Autodesk Fusion 360 part; units mm, degrees
(part 6 of 25)
  arc A2041 (23.4513, 13.1318) -> (23.4513, 13.1826) centre (23.4513, 13.1572) ccw
  line L640 (23.4513, 12.5081) -> (23.1267, 12.5081)
  arc A2042 (23.1521, 13.1572) -> (23.1013, 13.1572) centre (23.1267, 13.1572) ccw
  arc A2043 (25.2656, 11.9888) -> (25.3164, 11.9888) centre (25.291, 11.9888) ccw
  arc A2044 (26.4688, 12.2484) -> (26.7285, 11.9888) centre (26.7285, 12.2485) ccw
  arc A2045 (25.9147, 11.9888) -> (25.9655, 11.9888) centre (25.9401, 11.9888) ccw
  arc A2046 (21.1404, 12.6633) -> (21.1404, 12.6125) centre (21.1404, 12.6379) ccw
  line L641 (22.131, 13.1572) -> (22.6503, 13.1572)
  line L642 (25.291, 13.1572) -> (25.9401, 11.9888)
  arc A2047 (23.1267, 12.5335) -> (23.1267, 12.4827) centre (23.1267, 12.5081) ccw
  arc A2048 (22.131, 13.1826) -> (22.131, 13.1318) centre (22.131, 13.1572) ccw
  line L643 (23.1267, 13.1572) -> (23.4513, 13.1572)
  arc A2049 (23.4513, 12.5081) -> (23.4513, 13.1572) centre (23.4513, 12.8327) ccw
  arc A2050 (22.1564, 13.1572) -> (22.1056, 13.1572) centre (22.131, 13.1572) ccw
  arc A2051 (24.822, 13.1318) -> (24.822, 13.1826) centre (24.822, 13.1572) ccw
  arc A2052 (57.8335, 39.6198) -> (57.8335, 39.569) centre (57.8335, 39.5944) ccw
  arc A2053 (27.9843, 11.9634) -> (27.9843, 12.0142) centre (27.9843, 11.9888) ccw
  arc A2054 (25.9655, 13.1572) -> (25.9147, 13.1572) centre (25.9401, 13.1572) ccw
  arc A2055 (23.5389, 12.5194) -> (23.4934, 12.4967) centre (23.5162, 12.5081) ccw
  arc A2056 (23.4513, 12.4827) -> (23.4513, 12.5335) centre (23.4513, 12.5081) ccw
  arc A2057 (23.4513, 12.5335) -> (23.4513, 12.4827) centre (23.4513, 12.5081) ccw
  arc A2058 (26.7285, 13.1318) -> (26.7285, 13.1826) centre (26.7285, 13.1572) ccw
  arc A2059 (22.5205, 12.6125) -> (22.5205, 12.6633) centre (22.5205, 12.6379) ccw
  line L644 (24.3027, 12.6379) -> (24.6922, 12.6379)
  arc A2060 (24.3027, 12.0142) -> (24.3027, 11.9634) centre (24.3027, 11.9888) ccw
  arc A2061 (24.6922, 12.6125) -> (24.6922, 12.6633) centre (24.6922, 12.6379) ccw
  arc A2062 (22.6503, 13.1318) -> (22.6503, 13.1826) centre (22.6503, 13.1572) ccw
  line L645 (22.6503, 11.9888) -> (22.131, 11.9888)
  line L646 (23.7758, 11.9888) -> (23.5162, 12.5081)
  arc A2063 (27.465, 12.0142) -> (27.465, 11.9634) centre (27.465, 11.9888) ccw
  line L647 (23.1267, 11.9888) -> (23.1267, 13.1572)
  line L648 (27.465, 11.9888) -> (27.465, 13.1572)
  line L649 (21.1404, 12.6379) -> (21.6597, 12.6379)
  arc A2064 (26.7285, 11.9634) -> (26.7285, 12.0142) centre (26.7285, 11.9888) ccw
  line L650 (22.131, 12.6379) -> (22.5205, 12.6379)
  arc A2065 (26.4942, 12.2484) -> (26.4434, 12.2484) centre (26.4688, 12.2484) ccw
  arc A2066 (27.4904, 13.1572) -> (27.4396, 13.1572) centre (27.465, 13.1572) ccw
  arc A2067 (26.7285, 12.0142) -> (26.7285, 11.9634) centre (26.7285, 11.9888) ccw
  line L651 (24.3027, 11.9888) -> (24.3027, 13.1572)
  line L652 (22.131, 11.9888) -> (22.131, 13.1572)
  arc A2068 (23.1013, 11.9888) -> (23.1521, 11.9888) centre (23.1267, 11.9888) ccw
  arc A2069 (24.3027, 12.6633) -> (24.3027, 12.6125) centre (24.3027, 12.6379) ccw
  arc A2070 (22.131, 12.6633) -> (22.131, 12.6125) centre (22.131, 12.6379) ccw
  arc A2071 (23.1267, 13.1826) -> (23.1267, 13.1318) centre (23.1267, 13.1572) ccw
  arc A2072 (22.131, 12.0142) -> (22.131, 11.9634) centre (22.131, 11.9888) ccw
  line L653 (57.8984, 39.0751) -> (57.8984, 39.0102)
  line L654 (24.822, 11.9888) -> (24.3027, 11.9888)
  arc A2073 (23.4513, 13.1826) -> (23.4513, 13.1318) centre (23.4513, 13.1572) ccw
  arc A2074 (22.6503, 11.9634) -> (22.6503, 12.0142) centre (22.6503, 11.9888) ccw
  arc A2075 (24.3281, 13.1572) -> (24.2773, 13.1572) centre (24.3027, 13.1572) ccw
  line L655 (27.9843, 11.9888) -> (27.465, 11.9888)
  arc A2076 (25.3132, 13.1695) -> (25.2688, 13.1449) centre (25.291, 13.1572) ccw
  line L656 (26.9881, 11.9888) -> (26.7285, 11.9888)
  arc A2077 (19.2984, 13.1826) -> (19.2984, 13.1318) centre (19.2984, 13.1572) ccw
  arc A2078 (22.1056, 11.9888) -> (22.1564, 11.9888) centre (22.131, 11.9888) ccw
  arc A2079 (23.7531, 11.9774) -> (23.7985, 12.0002) centre (23.7758, 11.9888) ccw
  line L657 (25.291, 11.9888) -> (25.291, 13.1572)
  arc A2080 (24.2773, 11.9888) -> (24.3281, 11.9888) centre (24.3027, 11.9888) ccw
  line L658 (24.3027, 13.1572) -> (24.822, 13.1572)
  arc A2081 (19.2984, 10.5777) -> (19.2984, 10.6285) centre (19.2984, 10.6031) ccw
  arc A2082 (21.3939, 10.0584) -> (21.3939, 10.1092) centre (21.3939, 10.0838) ccw
  arc A2083 (20.0838, 10.3434) -> (20.033, 10.3434) centre (20.0584, 10.3434) ccw
  arc A2084 (21.0693, 11.2776) -> (21.0693, 11.2268) centre (21.0693, 11.2522) ccw
  line L659 (26.4688, 12.2484) -> (26.4688, 12.8976)
  arc A2085 (27.4396, 11.9888) -> (27.4904, 11.9888) centre (27.465, 11.9888) ccw
  arc A2086 (19.2984, 10.6031) -> (19.2984, 11.2522) centre (19.2984, 10.9277) ccw
  line L660 (21.0693, 10.0838) -> (21.0693, 11.2522)
  arc A2087 (21.0439, 10.0838) -> (21.0947, 10.0838) centre (21.0693, 10.0838) ccw
  line L661 (27.465, 12.6379) -> (27.8545, 12.6379)
  arc A2088 (26.4942, 12.8976) -> (26.4434, 12.8976) centre (26.4688, 12.8976) ccw
  arc A2089 (19.2984, 10.6285) -> (19.2984, 10.5777) centre (19.2984, 10.6031) ccw
  arc A2090 (27.465, 13.1826) -> (27.465, 13.1318) centre (27.465, 13.1572) ccw
  line L662 (21.0693, 10.7329) -> (21.3939, 10.7329)
  arc A2091 (20.0838, 10.9926) -> (20.033, 10.9926) centre (20.0584, 10.9926) ccw
  arc A2092 (21.3939, 11.2268) -> (21.3939, 11.2776) centre (21.3939, 11.2522) ccw
  arc A2093 (21.3939, 11.2776) -> (21.3939, 11.2268) centre (21.3939, 11.2522) ccw
  arc A2094 (21.3939, 10.1092) -> (21.3939, 10.0584) centre (21.3939, 10.0838) ccw
  arc A2095 (21.3939, 10.7583) -> (21.3939, 10.7075) centre (21.3939, 10.7329) ccw
  arc A2096 (26.4434, 12.2484) -> (26.4942, 12.2484) centre (26.4688, 12.2484) ccw
  arc A2097 (18.9738, 10.6285) -> (18.9738, 10.5777) centre (18.9738, 10.6031) ccw
  arc A2098 (20.3181, 11.2268) -> (20.3181, 11.2776) centre (20.3181, 11.2522) ccw
  arc A2099 (21.3939, 10.7075) -> (21.3939, 10.7583) centre (21.3939, 10.7329) ccw
  arc A2100 (20.3181, 11.2522) -> (20.0584, 10.9926) centre (20.3181, 10.9925) ccw
  arc A2101 (26.7285, 13.1572) -> (26.4688, 12.8976) centre (26.7285, 12.8975) ccw
  arc A2102 (27.465, 12.6633) -> (27.465, 12.6125) centre (27.465, 12.6379) ccw
  line L663 (21.0693, 11.2522) -> (21.3939, 11.2522)
  arc A2103 (21.0693, 10.7583) -> (21.0693, 10.7075) centre (21.0693, 10.7329) ccw
  arc A2104 (20.5777, 11.2268) -> (20.5777, 11.2776) centre (20.5777, 11.2522) ccw
  arc A2105 (19.2984, 11.2268) -> (19.2984, 11.2776) centre (19.2984, 11.2522) ccw
  line L664 (20.5777, 10.0838) -> (20.3181, 10.0838)
  arc A2106 (20.033, 10.9926) -> (20.0838, 10.9926) centre (20.0584, 10.9926) ccw
  arc A2107 (26.4434, 12.8976) -> (26.4942, 12.8976) centre (26.4688, 12.8976) ccw
  arc A2108 (20.3181, 10.1092) -> (20.3181, 10.0584) centre (20.3181, 10.0838) ccw
  arc A2109 (20.3181, 10.0584) -> (20.3181, 10.1092) centre (20.3181, 10.0838) ccw
  arc A2110 (20.5777, 10.0584) -> (20.5777, 10.1092) centre (20.5777, 10.0838) ccw
  arc A2111 (21.0947, 11.2522) -> (21.0439, 11.2522) centre (21.0693, 11.2522) ccw
  line L665 (19.2984, 10.6031) -> (18.9738, 10.6031)
  arc A2112 (26.9881, 13.1318) -> (26.9881, 13.1826) centre (26.9881, 13.1572) ccw
  line L666 (27.465, 13.1572) -> (27.9843, 13.1572)
  arc A2113 (21.0693, 10.1092) -> (21.0693, 10.0584) centre (21.0693, 10.0838) ccw
  arc A2114 (21.3939, 10.7583) -> (21.3939, 10.7075) centre (21.3939, 10.7329) ccw
  line L667 (20.0584, 10.3434) -> (20.0584, 10.9926)
  arc A2115 (20.0584, 10.3434) -> (20.3181, 10.0838) centre (20.3181, 10.3435) ccw
  arc A2116 (21.3939, 10.0838) -> (21.3939, 10.7329) centre (21.3939, 10.4084) ccw
  line L668 (21.3939, 10.0838) -> (21.0693, 10.0838)
  line L669 (26.7285, 13.1572) -> (26.9881, 13.1572)
  line L670 (18.9738, 11.2522) -> (19.2984, 11.2522)
  line L671 (25.9401, 11.9888) -> (25.9401, 13.1572)
  arc A2117 (20.3181, 11.2776) -> (20.3181, 11.2268) centre (20.3181, 11.2522) ccw
  arc A2118 (18.9992, 11.2522) -> (18.9484, 11.2522) centre (18.9738, 11.2522) ccw
  arc A2119 (18.9484, 10.0838) -> (18.9992, 10.0838) centre (18.9738, 10.0838) ccw
  line L672 (18.9738, 10.0838) -> (18.9738, 11.2522)
  arc A2120 (20.033, 10.3434) -> (20.0838, 10.3434) centre (20.0584, 10.3434) ccw
  arc A2121 (19.2984, 11.2776) -> (19.2984, 11.2268) centre (19.2984, 11.2522) ccw
  line L673 (20.3181, 11.2522) -> (20.5777, 11.2522)
  arc A2122 (18.9738, 11.2776) -> (18.9738, 11.2268) centre (18.9738, 11.2522) ccw
  arc A2123 (22.6314, 42.8554) -> (22.6822, 42.8554) centre (22.6568, 42.8554) ccw
  arc A2124 (21.3939, 10.7329) -> (21.3939, 11.2522) centre (21.3939, 10.9926) ccw
  arc A2125 (27.8545, 12.6125) -> (27.8545, 12.6633) centre (27.8545, 12.6379) ccw
  arc A2126 (27.9843, 13.1318) -> (27.9843, 13.1826) centre (27.9843, 13.1572) ccw
  arc A2127 (23.1761, 42.5704) -> (23.1761, 42.6212) centre (23.1761, 42.5958) ccw
  arc A2128 (22.9164, 43.7388) -> (22.9164, 43.7896) centre (22.9164, 43.7642) ccw
  arc A2129 (22.9814, 41.1988) -> (22.9814, 41.2496) centre (22.9814, 41.2242) ccw
  arc A2130 (22.6568, 41.2496) -> (22.6568, 41.1988) centre (22.6568, 41.2242) ccw
  arc A2131 (22.6568, 37.5412) -> (22.6568, 37.4904) centre (22.6568, 37.5158) ccw
  arc A2132 (22.6568, 40.0812) -> (22.6568, 40.0304) centre (22.6568, 40.0558) ccw
  arc A2133 (22.9814, 40.7303) -> (22.9814, 40.6795) centre (22.9814, 40.7049) ccw
  arc A2134 (22.6822, 43.5046) -> (22.6314, 43.5046) centre (22.6568, 43.5046) ccw
  line L674 (22.9164, 43.7642) -> (23.1761, 43.7642)
  arc A2135 (23.1761, 37.4904) -> (23.1761, 37.5412) centre (23.1761, 37.5158) ccw
  arc A2136 (22.6568, 38.1903) -> (22.6568, 38.1395) centre (22.6568, 38.1649) ccw
  arc A2137 (22.6822, 42.8554) -> (22.6314, 42.8554) centre (22.6568, 42.8554) ccw
  line L675 (22.6568, 37.5158) -> (22.6568, 38.6842)
  arc A2138 (72.1043, 51.3715) -> (72.0408, 51.3715) centre (72.0726, 51.3715) ccw
  arc A2139 (23.1761, 38.6588) -> (23.1761, 38.7096) centre (23.1761, 38.6842) ccw
  arc A2140 (72.3265, 52.2287) -> (72.3265, 52.2923) centre (72.3265, 52.2605) ccw
  line L676 (72.5805, 51.1175) -> (72.3265, 51.1175)
  arc A2141 (72.3265, 52.2605) -> (72.0725, 52.0065) centre (72.3265, 52.0065) ccw
  arc A2142 (73.0287, 51.1493) -> (73.0287, 51.0857) centre (73.0287, 51.1175) ccw
  line L677 (72.0725, 51.3715) -> (72.0725, 52.0065)
  arc A2143 (22.6314, 37.5158) -> (22.6822, 37.5158) centre (22.6568, 37.5158) ccw
  arc A2144 (72.0408, 52.0065) -> (72.1043, 52.0065) centre (72.0726, 52.0065) ccw
  arc A2145 (72.5805, 52.2287) -> (72.5805, 52.2923) centre (72.5805, 52.2605) ccw
  arc A2146 (73.6637, 51.0857) -> (73.6637, 51.1493) centre (73.6637, 51.1175) ccw
  arc A2147 (73.3145, 51.1175) -> (73.378, 51.1175) centre (73.3462, 51.1175) ccw
  arc A2148 (73.378, 52.2605) -> (73.3145, 52.2605) centre (73.3462, 52.2605) ccw
  arc A2149 (22.9164, 42.5704) -> (22.9164, 42.6212) centre (22.9164, 42.5958) ccw
  line L678 (22.6568, 40.7049) -> (22.9814, 40.7049)
  arc A2150 (22.9814, 40.0558) -> (22.9814, 40.7049) centre (22.9814, 40.3803) ccw
  line L679 (22.6568, 40.0558) -> (22.6568, 41.2242)
  line L680 (22.6568, 38.6842) -> (23.1761, 38.6842)
  arc A2151 (22.6822, 38.6842) -> (22.6314, 38.6842) centre (22.6568, 38.6842) ccw
  arc A2152 (72.1043, 52.0065) -> (72.0408, 52.0065) centre (72.0726, 52.0065) ccw
  arc A2153 (22.9814, 41.2496) -> (22.9814, 41.1988) centre (22.9814, 41.2242) ccw
  arc A2154 (22.9814, 40.7049) -> (22.9814, 41.2242) centre (22.9814, 40.9646) ccw
  arc A2155 (72.3265, 52.2923) -> (72.3265, 52.2287) centre (72.3265, 52.2605) ccw
  line L681 (22.6568, 38.1649) -> (23.0463, 38.1649)
  line L682 (73.0287, 52.0065) -> (73.3462, 52.2605)
  line L683 (23.1761, 42.5958) -> (22.9164, 42.5958)
  arc A2156 (22.9164, 42.6212) -> (22.9164, 42.5704) centre (22.9164, 42.5958) ccw
  arc A2157 (22.6314, 40.0558) -> (22.6822, 40.0558) centre (22.6568, 40.0558) ccw
  arc A2158 (22.6314, 43.5046) -> (22.6822, 43.5046) centre (22.6568, 43.5046) ccw
  arc A2159 (72.3265, 51.1493) -> (72.3265, 51.0857) centre (72.3265, 51.1175) ccw
  arc A2160 (72.5805, 51.0857) -> (72.5805, 51.1493) centre (72.5805, 51.1175) ccw
  line L684 (22.6568, 42.8554) -> (22.6568, 43.5046)
  arc A2161 (22.6568, 42.8554) -> (22.9164, 42.5958) centre (22.9164, 42.8554) ccw
  arc A2162 (22.9164, 43.7896) -> (22.9164, 43.7388) centre (22.9164, 43.7642) ccw
  arc A2163 (22.6568, 38.7096) -> (22.6568, 38.6588) centre (22.6568, 38.6842) ccw
  arc A2164 (22.6822, 41.2242) -> (22.6314, 41.2242) centre (22.6568, 41.2242) ccw
  line L685 (73.3462, 52.2605) -> (73.3462, 51.1175)
  arc A2165 (23.0463, 38.1395) -> (23.0463, 38.1903) centre (23.0463, 38.1649) ccw
  arc A2166 (72.0725, 51.3715) -> (72.3265, 51.1175) centre (72.3265, 51.3715) ccw
  arc A2167 (22.9814, 40.0812) -> (22.9814, 40.0304) centre (22.9814, 40.0558) ccw
  line L686 (22.9814, 40.0558) -> (22.6568, 40.0558)
  arc A2168 (22.9814, 40.7303) -> (22.9814, 40.6795) centre (22.9814, 40.7049) ccw
  line L687 (23.1761, 37.5158) -> (22.6568, 37.5158)
  arc A2169 (22.9164, 43.7642) -> (22.6568, 43.5046) centre (22.9164, 43.5046) ccw
  arc A2170 (23.1761, 43.7388) -> (23.1761, 43.7896) centre (23.1761, 43.7642) ccw
  arc A2171 (22.6568, 40.7303) -> (22.6568, 40.6795) centre (22.6568, 40.7049) ccw
  arc A2172 (22.9814, 40.0304) -> (22.9814, 40.0812) centre (22.9814, 40.0558) ccw
  line L688 (22.6568, 41.2242) -> (22.9814, 41.2242)
  arc A2173 (72.0408, 51.3715) -> (72.1043, 51.3715) centre (72.0726, 51.3715) ccw
  arc A2174 (22.9814, 40.6795) -> (22.9814, 40.7303) centre (22.9814, 40.7049) ccw
  arc A2175 (73.3661, 52.2357) -> (73.3264, 52.2853) centre (73.3463, 52.2605) ccw
  arc A2176 (73.0089, 52.0313) -> (73.0486, 51.9817) centre (73.0288, 52.0065) ccw
  line L689 (72.3265, 52.2605) -> (72.5805, 52.2605)
  arc A2177 (55.0545, 20.5422) -> (55.0545, 20.4788) centre (55.0545, 20.5105) ccw
  arc A2178 (56.106, 20.5105) -> (55.7567, 20.2565) centre (56.106, 20.1434) ccw
  arc A2179 (11.9697, 38.608) -> (12.0333, 38.608) centre (12.0015, 38.608) ccw
  arc A2180 (11.176, 38.9255) -> (10.8585, 38.608) centre (11.176, 38.608) ccw
  arc A2181 (11.9697, 38.2905) -> (12.0333, 38.2905) centre (12.0015, 38.2905) ccw
  arc A2182 (56.3917, 19.3358) -> (56.3917, 19.3992) centre (56.3917, 19.3675) ccw
  line L690 (12.0015, 38.2905) -> (10.8585, 38.2905)
  arc A2183 (11.1443, 40.0748) -> (11.1443, 40.1384) centre (11.1443, 40.1066) ccw
  arc A2184 (11.3871, 40.0355) -> (11.3459, 39.9872) centre (11.3665, 40.0114) ccw
  arc A2185 (12.0015, 38.608) -> (11.684, 38.9255) centre (11.684, 38.608) ccw
  arc A2186 (11.176, 38.8937) -> (11.176, 38.9573) centre (11.176, 38.9255) ccw
  arc A2187 (11.684, 38.9573) -> (11.684, 38.8937) centre (11.684, 38.9255) ccw
  line L691 (56.2965, 20.0025) -> (55.7567, 19.3675)
  arc A2188 (56.36, 20.2248) -> (56.4235, 20.2248) centre (56.3918, 20.2248) ccw
  arc A2189 (55.0545, 19.3358) -> (55.0545, 19.3992) centre (55.0545, 19.3675) ccw
  arc A2190 (55.3085, 19.3358) -> (55.3085, 19.3992) centre (55.3085, 19.3675) ccw
  arc A2191 (55.0545, 20.5105) -> (54.8005, 20.2565) centre (55.0545, 20.2565) ccw
  arc A2192 (55.7325, 19.3881) -> (55.7809, 19.3469) centre (55.7567, 19.3675) ccw
  arc A2193 (54.8323, 19.6215) -> (54.7687, 19.6215) centre (54.8005, 19.6215) ccw
  arc A2194 (56.106, 20.5422) -> (56.106, 20.4788) centre (56.106, 20.5105) ccw
  arc A2195 (55.0545, 19.3992) -> (55.0545, 19.3358) centre (55.0545, 19.3675) ccw
  arc A2196 (56.2746, 20.0255) -> (56.3184, 19.9795) centre (56.2965, 20.0025) ccw
  arc A2197 (56.4235, 20.2248) -> (56.36, 20.2247) centre (56.3918, 20.2248) ccw
  line L692 (54.8005, 19.6215) -> (54.8005, 20.2565)
  arc A2198 (54.7687, 19.6215) -> (54.8323, 19.6215) centre (54.8005, 19.6215) ccw
  arc A2199 (12.0015, 38.2587) -> (12.0015, 38.3223) centre (12.0015, 38.2905) ccw
  arc A2200 (55.0545, 20.4788) -> (55.0545, 20.5422) centre (55.0545, 20.5105) ccw
  arc A2201 (10.8585, 38.3223) -> (10.8585, 38.2587) centre (10.8585, 38.2905) ccw
  arc A2202 (11.176, 38.9573) -> (11.176, 38.8937) centre (11.176, 38.9255) ccw
  arc A2203 (11.1442, 40.1383) -> (11.1443, 40.0749) centre (11.1442, 40.1066) ccw
  arc A2204 (11.3665, 40.0114) -> (11.1443, 40.1066) centre (11.1444, 39.7998) ccw
  line L693 (55.0545, 20.5105) -> (55.3085, 20.5105)
  arc A2205 (54.7687, 20.2565) -> (54.8323, 20.2565) centre (54.8005, 20.2565) ccw
  arc A2206 (72.3265, 51.0857) -> (72.3265, 51.1493) centre (72.3265, 51.1175) ccw
  arc A2207 (56.2965, 20.0025) -> (56.3917, 20.2248) centre (56.0848, 20.2247) ccw
  arc A2208 (54.8005, 19.6215) -> (55.0545, 19.3675) centre (55.0545, 19.6215) ccw
  arc A2209 (55.7567, 19.3992) -> (55.7567, 19.3358) centre (55.7567, 19.3675) ccw
  arc A2210 (56.3207, 19.9819) -> (56.2723, 20.0231) centre (56.2965, 20.0025) ccw
  line L694 (12.0015, 39.4716) -> (12.0015, 40.1066)
  line L695 (10.8585, 38.2905) -> (10.8585, 38.608)
  arc A2211 (12.0333, 40.1066) -> (11.9697, 40.1066) centre (12.0015, 40.1066) ccw
  arc A2212 (10.8268, 39.8209) -> (10.8903, 39.8209) centre (10.8586, 39.8209) ccw
  arc A2213 (55.3085, 20.4788) -> (55.3085, 20.5422) centre (55.3085, 20.5105) ccw
  arc A2214 (10.8268, 38.608) -> (10.8903, 38.608) centre (10.8586, 38.608) ccw
  line L696 (55.7567, 19.3675) -> (56.3917, 19.3675)
  arc A2215 (11.1443, 40.1066) -> (10.8585, 39.8209) centre (11.1443, 39.8208) ccw
  arc A2216 (56.3917, 20.2248) -> (56.106, 20.5105) centre (56.106, 20.2248) ccw
  arc A2217 (43.9774, 31.3303) -> (44.017, 31.2807) centre (43.9972, 31.3055) ccw
  arc A2218 (10.8903, 38.608) -> (10.8268, 38.608) centre (10.8586, 38.608) ccw
  arc A2219 (56.106, 20.4788) -> (56.106, 20.5422) centre (56.106, 20.5105) ccw
  arc A2220 (11.684, 38.8937) -> (11.684, 38.9573) centre (11.684, 38.9255) ccw
  arc A2221 (12.0333, 38.608) -> (11.9697, 38.608) centre (12.0015, 38.608) ccw
  line L697 (55.3085, 19.3675) -> (55.0545, 19.3675)
  arc A2222 (11.3435, 39.9895) -> (11.3895, 40.0332) centre (11.3665, 40.0114) ccw
  arc A2223 (54.8323, 20.2565) -> (54.7687, 20.2565) centre (54.8005, 20.2565) ccw
  line L698 (11.176, 38.9255) -> (11.684, 38.9255)
  line L699 (73.0287, 51.1175) -> (73.6637, 51.1175)
  arc A2224 (11.9697, 39.4716) -> (12.0333, 39.4716) centre (12.0015, 39.4716) ccw
  line L700 (11.3665, 40.0114) -> (12.0015, 39.4716)
  arc A2225 (11.1027, 39.4414) -> (11.1223, 39.5018) centre (11.1125, 39.4716) ccw
  arc A2226 (10.8903, 39.8208) -> (10.8268, 39.8209) centre (10.8586, 39.8209) ccw
  arc A2227 (10.8268, 38.2905) -> (10.8903, 38.2905) centre (10.8586, 38.2905) ccw
  arc A2228 (55.7265, 20.2663) -> (55.7869, 20.2467) centre (55.7567, 20.2565) ccw
  line L701 (12.0015, 38.608) -> (12.0015, 38.2905)
  line L702 (71.2799, 44.5135) -> (71.2799, 44.0055)
  line L703 (42.3545, 30.4165) -> (42.1005, 30.9245)
  arc A2229 (42.037, 31.5278) -> (42.037, 31.5912) centre (42.037, 31.5595) ccw
  line L704 (42.037, 30.9245) -> (41.7195, 30.9245)
  arc A2230 (24.2264, 26.0668) -> (24.2264, 26.1303) centre (24.2264, 26.0985) ccw
  arc A2231 (41.7195, 30.9563) -> (41.7195, 30.8928) centre (41.7195, 30.9246) ccw
  arc A2232 (23.0505, 24.9555) -> (23.3045, 25.2095) centre (23.0505, 25.2095) ccw
  arc A2233 (23.0505, 24.9238) -> (23.0505, 24.9872) centre (23.0505, 24.9555) ccw
  arc A2234 (23.9724, 25.6223) -> (23.9724, 25.5588) centre (23.9724, 25.5906) ccw
  arc A2235 (43.4892, 30.3848) -> (43.4892, 30.4483) centre (43.4892, 30.4166) ccw
  line L705 (23.8454, 26.0985) -> (24.2264, 26.0985)
  arc A2236 (24.1629, 25.6223) -> (24.1629, 25.5588) centre (24.1629, 25.5906) ccw
  arc A2237 (41.7513, 31.5595) -> (41.6878, 31.5595) centre (41.7196, 31.5595) ccw
  arc A2238 (22.9235, 24.9872) -> (22.9235, 24.9238) centre (22.9235, 24.9555) ccw
  arc A2239 (24.1629, 24.9872) -> (24.1629, 24.9238) centre (24.1629, 24.9555) ccw
  arc A2240 (71.1199, 45.1398) -> (71.0588, 45.1572) centre (71.0894, 45.1485) ccw
  arc A2241 (24.2264, 25.5588) -> (24.2264, 25.6223) centre (24.2264, 25.5906) ccw
  line L706 (70.2945, 45.1485) -> (70.2945, 44.2595)
  line L707 (41.7195, 30.4165) -> (41.7195, 31.5595)
  arc A2242 (70.3263, 45.1485) -> (70.2627, 45.1485) centre (70.2945, 45.1485) ccw
  arc A2243 (70.3263, 44.2595) -> (70.2627, 44.2595) centre (70.2945, 44.2595) ccw
  line L708 (23.0505, 24.9555) -> (22.9235, 24.9555)
  line L709 (70.2945, 32.4485) -> (70.2945, 31.5595)
  line L710 (71.0894, 45.1485) -> (70.8354, 44.2595)
  arc A2244 (43.1915, 31.5347) -> (43.1519, 31.5843) centre (43.1717, 31.5595) ccw
  arc A2245 (10.8585, 39.8209) -> (11.1125, 39.4716) centre (11.2256, 39.8209) ccw
  arc A2246 (43.2035, 31.5595) -> (43.14, 31.5595) centre (43.1717, 31.5595) ccw
  line L711 (42.8542, 31.3055) -> (43.1717, 31.5595)
  arc A2247 (42.037, 30.8928) -> (42.037, 30.9563) centre (42.037, 30.9246) ccw
  arc A2248 (42.037, 30.9563) -> (42.037, 30.8928) centre (42.037, 30.9246) ccw
  arc A2249 (23.3362, 25.2095) -> (23.2728, 25.2095) centre (23.3045, 25.2095) ccw
  arc A2250 (41.7195, 31.5912) -> (41.7195, 31.5278) centre (41.7195, 31.5595) ccw
  arc A2251 (42.8542, 30.4483) -> (42.8542, 30.3848) centre (42.8542, 30.4166) ccw
  arc A2252 (23.8454, 26.1303) -> (23.8454, 26.0668) centre (23.8454, 26.0985) ccw
  arc A2253 (24.2264, 26.1303) -> (24.2264, 26.0668) centre (24.2264, 26.0985) ccw
  arc A2254 (23.3362, 26.0985) -> (23.2728, 26.0985) centre (23.3045, 26.0985) ccw
  arc A2255 (42.037, 30.9245) -> (42.037, 31.5595) centre (42.037, 31.242) ccw
  arc A2256 (42.037, 31.5912) -> (42.037, 31.5278) centre (42.037, 31.5595) ccw
  line L712 (43.9972, 31.3055) -> (44.3147, 31.5595)
  line L713 (23.8454, 24.9555) -> (24.1629, 24.9555)
  arc A2257 (24.1629, 24.9238) -> (24.1629, 24.9872) centre (24.1629, 24.9555) ccw
  line L714 (23.3045, 26.0985) -> (23.3045, 25.2095)
  line L715 (43.1717, 31.5595) -> (43.1717, 30.4165)
  line L716 (42.8542, 30.4165) -> (43.4892, 30.4165)
  arc A2258 (42.8344, 31.3303) -> (42.874, 31.2807) centre (42.8542, 31.3055) ccw
  arc A2259 (42.3261, 30.4023) -> (42.3829, 30.4307) centre (42.3545, 30.4165) ccw
  arc A2260 (42.1289, 30.9387) -> (42.0721, 30.9103) centre (42.1005, 30.9245) ccw
  arc A2261 (23.0505, 24.9872) -> (23.0505, 24.9238) centre (23.0505, 24.9555) ccw
  arc A2262 (44.3465, 31.5595) -> (44.283, 31.5595) centre (44.3147, 31.5595) ccw
  arc A2263 (24.1629, 24.9555) -> (24.1629, 25.5905) centre (24.1629, 25.273) ccw
  arc A2264 (44.3345, 31.5347) -> (44.2949, 31.5843) centre (44.3147, 31.5595) ccw
  arc A2265 (41.6878, 30.4165) -> (41.7513, 30.4165) centre (41.7196, 30.4165) ccw
  arc A2266 (24.2264, 25.6223) -> (24.2264, 25.5588) centre (24.2264, 25.5906) ccw
  arc A2267 (24.2264, 25.5905) -> (24.2264, 26.0985) centre (24.2264, 25.8445) ccw
  line L717 (41.7195, 31.5595) -> (42.037, 31.5595)
  arc A2268 (11.9809, 39.4474) -> (12.0221, 39.4958) centre (12.0015, 39.4716) ccw
  arc A2269 (43.14, 30.4165) -> (43.2035, 30.4165) centre (43.1717, 30.4165) ccw
  arc A2270 (71.2481, 44.0055) -> (71.3116, 44.0055) centre (71.2798, 44.0055) ccw
  arc A2271 (23.8454, 24.9872) -> (23.8454, 24.9238) centre (23.8454, 24.9555) ccw
  arc A2272 (71.4704, 44.2278) -> (71.4704, 44.2913) centre (71.4704, 44.2596) ccw
  arc A2273 (44.283, 30.4165) -> (44.3465, 30.4165) centre (44.3147, 30.4165) ccw
  line L718 (24.2264, 25.5905) -> (23.9724, 25.5905)
  arc A2274 (23.2728, 25.2095) -> (23.3362, 25.2095) centre (23.3045, 25.2095) ccw
  arc A2275 (70.0405, 44.0373) -> (70.0405, 43.9738) centre (70.0405, 44.0055) ccw
  arc A2276 (56.1034, 43.8468) -> (56.1034, 43.9103) centre (56.1034, 43.8786) ccw
  arc A2277 (55.5636, 43.053) -> (55.6271, 43.053) centre (55.5954, 43.053) ccw
  arc A2278 (56.2621, 43.1165) -> (56.1986, 43.1165) centre (56.2304, 43.1165) ccw
  arc A2279 (56.2304, 43.1165) -> (55.9764, 43.3705) centre (55.9764, 43.1165) ccw
  arc A2280 (55.6271, 43.053) -> (55.5636, 43.053) centre (55.5954, 43.053) ccw
  arc A2281 (70.0405, 43.9738) -> (70.0405, 44.0373) centre (70.0405, 44.0055) ccw
  line L719 (55.0545, 43.8785) -> (55.0545, 42.9895)
  arc A2282 (71.2164, 31.3055) -> (71.4704, 31.5595) centre (71.2164, 31.5595) ccw
  arc A2283 (55.9764, 43.3387) -> (55.9764, 43.4023) centre (55.9764, 43.3705) ccw
  arc A2284 (70.0405, 44.0055) -> (70.2945, 44.2595) centre (70.0405, 44.2595) ccw
  arc A2285 (70.8048, 44.2682) -> (70.8659, 44.2508) centre (70.8354, 44.2595) ccw
  line L720 (70.8354, 31.9405) -> (70.8354, 32.4485)
  line L721 (70.8354, 44.2595) -> (71.4704, 44.2595)
  arc A2286 (70.3263, 32.4485) -> (70.2627, 32.4485) centre (70.2945, 32.4485) ccw
  line L722 (70.8354, 31.3055) -> (71.2164, 31.3055)
  line L723 (70.8354, 32.4485) -> (71.4704, 32.4485)
  arc A2287 (71.2164, 31.9088) -> (71.2164, 31.9722) centre (71.2164, 31.9405) ccw
  arc A2288 (70.3263, 31.5595) -> (70.2627, 31.5595) centre (70.2945, 31.5595) ccw
  arc A2289 (71.4704, 31.6865) -> (71.2164, 31.9405) centre (71.2164, 31.6865) ccw
  arc A2290 (71.4704, 32.4168) -> (71.4704, 32.4803) centre (71.4704, 32.4486) ccw
  line L724 (70.0405, 31.3055) -> (69.9135, 31.3055)
  arc A2291 (70.8036, 31.9405) -> (70.8671, 31.9405) centre (70.8354, 31.9405) ccw
  arc A2292 (70.8354, 44.2913) -> (70.8354, 44.2278) centre (70.8354, 44.2596) ccw
  arc A2293 (70.0405, 31.2738) -> (70.0405, 31.3373) centre (70.0405, 31.3056) ccw
  arc A2294 (71.4386, 31.6865) -> (71.5021, 31.6865) centre (71.4703, 31.6865) ccw
  arc A2295 (55.5954, 43.053) -> (56.2304, 43.053) centre (55.9129, 43.053) ccw
  line L725 (30.2566, 39.8145) -> (30.2566, 38.9255)
  line L726 (55.5954, 43.053) -> (55.5954, 43.3705)
  arc A2296 (56.1986, 43.053) -> (56.2621, 43.053) centre (56.2304, 43.053) ccw
  arc A2297 (55.0228, 42.9895) -> (55.0863, 42.9895) centre (55.0546, 42.9895) ccw
  arc A2298 (56.2621, 43.053) -> (56.1986, 43.053) centre (56.2304, 43.053) ccw
  arc A2299 (55.5954, 43.4023) -> (55.5954, 43.3387) centre (55.5954, 43.3705) ccw
  arc A2300 (71.3116, 44.5135) -> (71.2481, 44.5135) centre (71.2798, 44.5135) ccw
  arc A2301 (55.5636, 43.3705) -> (55.6271, 43.3705) centre (55.5954, 43.3705) ccw
  arc A2302 (54.8005, 42.7673) -> (54.8005, 42.7037) centre (54.8005, 42.7355) ccw
  arc A2303 (70.2627, 44.2595) -> (70.3263, 44.2595) centre (70.2945, 44.2595) ccw
  arc A2304 (71.2164, 31.2738) -> (71.2164, 31.3373) centre (71.2164, 31.3056) ccw
  arc A2305 (70.8671, 32.4485) -> (70.8036, 32.4485) centre (70.8354, 32.4485) ccw
  arc A2306 (71.4386, 31.5595) -> (71.5021, 31.5595) centre (71.4703, 31.5595) ccw
  arc A2307 (70.0405, 31.3373) -> (70.0405, 31.2738) centre (70.0405, 31.3056) ccw
  arc A2308 (71.2164, 31.3373) -> (71.2164, 31.2738) centre (71.2164, 31.3056) ccw
  arc A2309 (70.8354, 32.4803) -> (70.8354, 32.4168) centre (70.8354, 32.4486) ccw
  arc A2310 (55.0863, 42.9895) -> (55.0228, 42.9895) centre (55.0546, 42.9895) ccw
  arc A2311 (69.9135, 44.0373) -> (69.9135, 43.9738) centre (69.9135, 44.0055) ccw
  line L727 (55.5954, 43.3705) -> (55.9764, 43.3705)
  arc A2312 (71.5021, 31.5595) -> (71.4386, 31.5595) centre (71.4703, 31.5595) ccw
  arc A2313 (55.6271, 43.3705) -> (55.5636, 43.3705) centre (55.5954, 43.3705) ccw
  arc A2314 (71.2164, 31.9722) -> (71.2164, 31.9088) centre (71.2164, 31.9405) ccw
  arc A2315 (69.9135, 31.3373) -> (69.9135, 31.2738) centre (69.9135, 31.3056) ccw
  line L728 (70.0405, 44.0055) -> (69.9135, 44.0055)
  line L729 (71.2164, 31.9405) -> (70.8354, 31.9405)
  arc A2316 (70.8354, 31.3373) -> (70.8354, 31.2738) centre (70.8354, 31.3056) ccw
  arc A2317 (54.8005, 42.7037) -> (54.8005, 42.7673) centre (54.8005, 42.7355) ccw
  arc A2318 (71.5021, 31.6865) -> (71.4386, 31.6865) centre (71.4703, 31.6865) ccw
  arc A2319 (56.1986, 43.1165) -> (56.2621, 43.1165) centre (56.2304, 43.1165) ccw
  arc A2320 (70.2627, 31.5595) -> (70.3263, 31.5595) centre (70.2945, 31.5595) ccw
  arc A2321 (55.0863, 43.8785) -> (55.0228, 43.8785) centre (55.0546, 43.8785) ccw
  arc A2322 (54.8005, 42.7355) -> (55.0545, 42.9895) centre (54.8005, 42.9895) ccw
  line L730 (71.4704, 31.5595) -> (71.4704, 31.6865)
  arc A2323 (70.8354, 31.9722) -> (70.8354, 31.9088) centre (70.8354, 31.9405) ccw
  arc A2324 (70.0405, 31.3055) -> (70.2945, 31.5595) centre (70.0405, 31.5595) ccw
  arc A2325 (55.9764, 43.4023) -> (55.9764, 43.3387) centre (55.9764, 43.3705) ccw
  arc A2326 (58.1354, 31.623) -> (58.7704, 31.623) centre (58.4529, 31.623) ccw
  line L731 (30.7975, 39.8145) -> (31.4325, 39.8145)
  arc A2327 (54.6735, 42.7673) -> (54.6735, 42.7037) centre (54.6735, 42.7355) ccw
  arc A2328 (30.2884, 39.8145) -> (30.2249, 39.8145) centre (30.2567, 39.8145) ccw
  arc A2329 (30.7658, 39.6875) -> (30.8293, 39.6875) centre (30.7976, 39.6875) ccw
  arc A2330 (57.3405, 31.3055) -> (57.5945, 31.5595) centre (57.3405, 31.5595) ccw
  arc A2331 (30.7975, 39.8463) -> (30.7975, 39.7828) centre (30.7975, 39.8145) ccw
  arc A2332 (57.3405, 31.3373) -> (57.3405, 31.2738) centre (57.3405, 31.3056) ccw
  arc A2333 (57.3405, 31.2738) -> (57.3405, 31.3373) centre (57.3405, 31.3056) ccw
  arc A2334 (58.7704, 31.623) -> (58.1354, 31.623) centre (58.4529, 31.623) ccw
  arc A2335 (31.0844, 38.68) -> (31.1456, 38.663) centre (31.115, 38.6715) ccw
  arc A2336 (31.4325, 39.7828) -> (31.4325, 39.8463) centre (31.4325, 39.8145) ccw
  line L732 (7.8105, 49.0855) -> (7.6835, 49.0855)
  arc A2337 (7.8105, 49.0855) -> (8.0645, 49.3395) centre (7.8105, 49.3395) ccw
  arc A2338 (58.7386, 31.623) -> (58.8021, 31.623) centre (58.7704, 31.623) ccw
  arc A2339 (58.8021, 31.623) -> (58.7386, 31.623) centre (58.7704, 31.623) ccw
  arc A2340 (57.6263, 32.4485) -> (57.5628, 32.4485) centre (57.5945, 32.4485) ccw
  arc A2341 (58.1036, 31.623) -> (58.1671, 31.623) centre (58.1354, 31.623) ccw
  arc A2342 (58.7386, 32.1945) -> (58.6751, 32.1945) centre (58.7069, 32.1945) ccw
  line L733 (31.4325, 39.8145) -> (31.115, 38.6715)
  arc A2343 (7.8105, 49.0538) -> (7.8105, 49.1173) centre (7.8105, 49.0856) ccw
  arc A2344 (9.2404, 49.5618) -> (9.2404, 49.6253) centre (9.2404, 49.5936) ccw
  arc A2345 (30.0026, 38.6715) -> (30.2566, 38.9255) centre (30.0026, 38.9255) ccw
  arc A2346 (29.8756, 38.7033) -> (29.8756, 38.6397) centre (29.8756, 38.6715) ccw
  arc A2347 (30.2249, 38.9255) -> (30.2884, 38.9255) centre (30.2567, 38.9255) ccw
  arc A2348 (7.8105, 49.1173) -> (7.8105, 49.0538) centre (7.8105, 49.0856) ccw
  arc A2349 (8.6371, 49.911) -> (8.5736, 49.911) centre (8.6054, 49.911) ccw
  arc A2350 (8.0963, 49.3395) -> (8.0328, 49.3395) centre (8.0646, 49.3395) ccw
  arc A2351 (58.6751, 32.1945) -> (58.7386, 32.1945) centre (58.7069, 32.1945) ccw
  line L734 (56.2304, 43.1165) -> (56.2304, 43.053)
  line L735 (9.2404, 49.5935) -> (8.8594, 49.5935)
  arc A2352 (58.1989, 32.1945) -> (58.7069, 32.1945) centre (58.4529, 32.1945) ccw
  line L736 (57.5945, 32.4485) -> (57.5945, 31.5595)
  arc A2353 (8.8594, 49.6253) -> (8.8594, 49.5618) centre (8.8594, 49.5936) ccw
  line L737 (8.0645, 50.2285) -> (8.0645, 49.3395)
  line L738 (30.7975, 39.6875) -> (30.7975, 39.8145)
  arc A2354 (8.6054, 49.8475) -> (8.8594, 49.5935) centre (8.8594, 49.8475) ccw
  arc A2355 (30.8293, 39.8145) -> (30.7658, 39.8145) centre (30.7976, 39.8145) ccw
  arc A2356 (57.2135, 31.3373) -> (57.2135, 31.2738) centre (57.2135, 31.3056) ccw
  arc A2357 (30.0026, 38.7033) -> (30.0026, 38.6397) centre (30.0026, 38.6715) ccw
  arc A2358 (30.2884, 38.9255) -> (30.2249, 38.9255) centre (30.2567, 38.9255) ccw
  arc A2359 (58.2306, 32.1945) -> (58.1671, 32.1945) centre (58.1989, 32.1945) ccw
  arc A2360 (58.1671, 31.623) -> (58.1036, 31.623) centre (58.1354, 31.623) ccw
  line L739 (54.8005, 42.7355) -> (54.6735, 42.7355)
  arc A2361 (8.0328, 49.3395) -> (8.0963, 49.3395) centre (8.0646, 49.3395) ccw
  arc A2362 (56.1034, 43.8785) -> (55.5954, 43.3705) centre (56.1034, 43.3705) ccw
  arc A2363 (57.6263, 31.5595) -> (57.5628, 31.5595) centre (57.5945, 31.5595) ccw
  arc A2364 (31.4631, 39.806) -> (31.4019, 39.823) centre (31.4325, 39.8145) ccw
  line L740 (30.0026, 38.6715) -> (29.8756, 38.6715)
  arc A2365 (7.6835, 49.1173) -> (7.6835, 49.0538) centre (7.6835, 49.0856) ccw
  arc A2366 (8.6371, 49.8475) -> (8.5736, 49.8475) centre (8.6054, 49.8475) ccw
  arc A2367 (8.8594, 49.5618) -> (8.8594, 49.6253) centre (8.8594, 49.5936) ccw
  arc A2368 (58.1671, 32.1945) -> (58.2306, 32.1945) centre (58.1989, 32.1945) ccw
  arc A2369 (57.5628, 31.5595) -> (57.6263, 31.5595) centre (57.5945, 31.5595) ccw
  line L741 (8.6054, 49.8475) -> (8.6054, 49.911)
  arc A2370 (8.0963, 50.2285) -> (8.0328, 50.2285) centre (8.0646, 50.2285) ccw
  line L742 (57.3405, 31.3055) -> (57.2135, 31.3055)
  arc A2371 (30.0026, 38.6397) -> (30.0026, 38.7033) centre (30.0026, 38.6715) ccw
  arc A2372 (58.7069, 32.1945) -> (58.1989, 32.1945) centre (58.4529, 32.1945) ccw
  arc A2373 (45.3073, 23.3045) -> (45.2437, 23.3045) centre (45.2755, 23.3045) ccw
  arc A2374 (31.8167, 35.0342) -> (31.8738, 35.0063) centre (31.8453, 35.0203) ccw
  arc A2375 (31.9722, 35.433) -> (31.9088, 35.433) centre (31.9405, 35.433) ccw
  arc A2376 (31.4308, 35.0305) -> (31.3707, 35.01) centre (31.4008, 35.0203) ccw
  line L743 (30.1625, 34.8615) -> (30.7975, 34.8615)
  arc A2377 (9.2721, 49.911) -> (9.2086, 49.911) centre (9.2404, 49.911) ccw
  arc A2378 (31.623, 35.9727) -> (31.623, 36.0363) centre (31.623, 36.0045) ccw
  arc A2379 (29.6534, 36.0045) -> (29.5899, 36.0045) centre (29.6217, 36.0045) ccw
  arc A2380 (31.3442, 35.1353) -> (31.3938, 35.0957) centre (31.369, 35.1155) ccw
  arc A2381 (9.2721, 49.5935) -> (9.2086, 49.5935) centre (9.2404, 49.5935) ccw
  arc A2382 (8.7324, 49.0855) -> (9.2404, 49.5935) centre (8.7324, 49.5935) ccw
  arc A2383 (29.6534, 35.1155) -> (29.5899, 35.1155) centre (29.6217, 35.1155) ccw
  arc A2384 (30.4998, 35.9797) -> (30.4602, 36.0293) centre (30.48, 36.0045) ccw
  arc A2385 (31.8738, 35.8597) -> (31.8167, 35.8318) centre (31.8453, 35.8457) ccw
  arc A2386 (31.9088, 35.433) -> (31.9722, 35.433) centre (31.9405, 35.433) ccw
  line L744 (29.6216, 36.0045) -> (29.6216, 35.1155)
  arc A2387 (29.5899, 35.1155) -> (29.6534, 35.1155) centre (29.6217, 35.1155) ccw
  arc A2388 (31.4008, 35.8458) -> (31.3055, 35.433) centre (32.2475, 35.4329) ccw
  line L745 (30.1625, 35.7505) -> (30.48, 36.0045)
  line L746 (45.0215, 22.1615) -> (44.8945, 22.1615)
  arc A2389 (31.623, 34.8615) -> (31.8453, 35.0203) centre (31.623, 35.0965) ccw
  arc A2390 (31.623, 36.0363) -> (31.623, 35.9727) centre (31.623, 36.0045) ccw
  arc A2391 (29.3676, 34.8297) -> (29.3676, 34.8933) centre (29.3676, 34.8615) ccw
  arc A2392 (30.1427, 35.7753) -> (30.1823, 35.7257) centre (30.1625, 35.7505) ccw
  arc A2393 (30.7975, 34.8297) -> (30.7975, 34.8933) centre (30.7975, 34.8615) ccw
  arc A2394 (31.3373, 35.433) -> (31.2738, 35.433) centre (31.3056, 35.433) ccw
  arc A2395 (31.3722, 35.0063) -> (31.4293, 35.0342) centre (31.4008, 35.0203) ccw
  arc A2396 (45.0215, 22.1615) -> (45.2755, 22.4155) centre (45.0215, 22.4155) ccw
  arc A2397 (44.8945, 22.1932) -> (44.8945, 22.1298) centre (44.8945, 22.1615) ccw
  arc A2398 (45.3073, 22.4155) -> (45.2437, 22.4155) centre (45.2755, 22.4155) ccw
  arc A2399 (31.8753, 35.01) -> (31.8152, 35.0305) centre (31.8453, 35.0203) ccw
  arc A2400 (31.8453, 35.0203) -> (31.9405, 35.433) centre (30.9988, 35.4329) ccw
  arc A2401 (31.623, 36.0045) -> (31.4008, 35.8458) centre (31.623, 35.7696) ccw
  arc A2402 (31.3055, 35.433) -> (31.4008, 35.0203) centre (32.2472, 35.4331) ccw
  arc A2403 (30.4483, 34.8615) -> (30.5117, 34.8615) centre (30.48, 34.8615) ccw
  arc A2404 (31.8152, 35.8355) -> (31.8753, 35.856) centre (31.8453, 35.8458) ccw
  line L747 (45.2755, 23.3045) -> (45.2755, 22.4155)
  arc A2405 (9.2086, 49.911) -> (9.2721, 49.911) centre (9.2404, 49.911) ccw
  arc A2406 (29.3676, 34.8615) -> (29.6216, 35.1155) centre (29.3676, 35.1155) ccw
  arc A2407 (9.2086, 49.5935) -> (9.2721, 49.5935) centre (9.2404, 49.5935) ccw
  arc A2408 (45.2437, 22.4155) -> (45.3073, 22.4155) centre (45.2755, 22.4155) ccw
  line L748 (31.369, 35.1155) -> (31.877, 35.7505)
  arc A2409 (31.4008, 35.0203) -> (31.623, 34.8615) centre (31.623, 35.0964) ccw
  arc A2410 (31.3707, 35.856) -> (31.4308, 35.8355) centre (31.4007, 35.8458) ccw
  arc A2411 (29.2406, 34.8933) -> (29.2406, 34.8297) centre (29.2406, 34.8615) ccw
  arc A2412 (31.623, 34.8933) -> (31.623, 34.8297) centre (31.623, 34.8615) ccw
  arc A2413 (8.5736, 49.8475) -> (8.6371, 49.8475) centre (8.6054, 49.8475) ccw
  arc A2414 (31.2738, 35.433) -> (31.3373, 35.433) centre (31.3056, 35.433) ccw
  arc A2415 (31.623, 34.8297) -> (31.623, 34.8933) centre (31.623, 34.8615) ccw
  arc A2416 (30.1625, 34.8933) -> (30.1625, 34.8297) centre (30.1625, 34.8615) ccw
  line L749 (30.48, 36.0045) -> (30.48, 34.8615)
  arc A2417 (9.2404, 49.911) -> (8.6054, 49.911) centre (8.9229, 49.911) ccw
  arc A2418 (29.3676, 34.8933) -> (29.3676, 34.8297) centre (29.3676, 34.8615) ccw
  arc A2419 (45.0215, 22.1932) -> (45.0215, 22.1298) centre (45.0215, 22.1615) ccw
  arc A2420 (31.4293, 35.8318) -> (31.3722, 35.8597) centre (31.4007, 35.8457) ccw
  arc A2421 (30.5117, 36.0045) -> (30.4483, 36.0045) centre (30.48, 36.0045) ccw
  arc A2422 (8.7324, 49.1173) -> (8.7324, 49.0538) centre (8.7324, 49.0856) ccw
  line L750 (9.2404, 49.911) -> (9.2404, 49.5935)
  line L751 (29.3676, 34.8615) -> (29.2406, 34.8615)
  arc A2423 (8.5736, 49.911) -> (8.6371, 49.911) centre (8.6054, 49.911) ccw
  arc A2424 (31.9405, 35.433) -> (31.8453, 35.8458) centre (30.9986, 35.4332) ccw
  line L752 (46.9594, 22.1615) -> (47.5944, 22.1615)
  arc A2425 (46.1537, 23.2797) -> (46.114, 23.3293) centre (46.1339, 23.3045) ccw
  arc A2426 (18.0199, 16.8275) -> (18.0199, 16.7005) centre (18.0199, 16.764) ccw
  arc A2427 (19.9488, 16.8051) -> (20.0456, 16.7229) centre (19.9972, 16.764) ccw
  arc A2428 (18.1822, 16.9898) -> (18.3092, 16.9898) centre (18.2457, 16.9898) ccw
  line L753 (20.477, 17.3284) -> (19.9972, 16.764)
  arc A2429 (19.1999, 17.78) -> (19.0729, 17.78) centre (19.1364, 17.78) ccw
  arc A2430 (31.8453, 35.8458) -> (31.623, 36.0045) centre (31.6231, 35.7696) ccw
  arc A2431 (20.5253, 17.2873) -> (20.4286, 17.3696) centre (20.477, 17.3284) ccw
  arc A2432 (47.2451, 22.1615) -> (47.3086, 22.1615) centre (47.2769, 22.1615) ccw
  arc A2433 (18.3092, 17.78) -> (18.1822, 17.78) centre (18.2457, 17.78) ccw
  line L754 (11.1718, 33.7058) -> (11.8209, 33.7058)
  arc A2434 (46.1021, 22.1615) -> (46.1656, 22.1615) centre (46.1339, 22.1615) ccw
  arc A2435 (20.3076, 17.78) -> (19.9972, 17.5542) centre (20.3076, 17.4537) ccw
  arc A2436 (19.9368, 17.5738) -> (20.0576, 17.5347) centre (19.9972, 17.5542) ccw
  line L755 (45.8164, 22.1615) -> (46.4514, 22.1615)
  arc A2437 (20.6251, 17.526) -> (20.4981, 17.526) centre (20.5616, 17.526) ccw
  arc A2438 (20.5616, 16.7005) -> (20.5616, 16.8275) centre (20.5616, 16.764) ccw
  arc A2439 (10.1092, 34.8742) -> (10.0584, 34.8742) centre (10.0838, 34.8742) ccw
  arc A2440 (18.8145, 17.6038) -> (18.8939, 17.5046) centre (18.8542, 17.5542) ccw
  arc A2441 (19.0729, 16.764) -> (19.1999, 16.764) centre (19.1364, 16.764) ccw
  arc A2442 (20.477, 17.3284) -> (20.5616, 17.526) centre (20.2888, 17.5259) ccw
  arc A2443 (18.3092, 16.9898) -> (18.1822, 16.9898) centre (18.2457, 16.9898) ccw
  arc A2444 (45.7965, 23.0753) -> (45.8362, 23.0257) centre (45.8163, 23.0505) ccw
  arc A2445 (17.907, 16.8275) -> (17.907, 16.7005) centre (17.907, 16.764) ccw
  arc A2446 (19.9972, 16.8275) -> (19.9972, 16.7005) centre (19.9972, 16.764) ccw
  arc A2447 (19.4186, 16.7005) -> (19.4186, 16.8275) centre (19.4186, 16.764) ccw
  line L756 (18.0199, 16.764) -> (17.907, 16.764)
  arc A2448 (19.1761, 17.7304) -> (19.0967, 17.8296) centre (19.1364, 17.78) ccw
  arc A2449 (11.4709, 33.7058) -> (11.5217, 33.7058) centre (11.4963, 33.7058) ccw
  line L757 (10.7329, 33.7058) -> (10.3434, 34.4198)
  arc A2450 (10.0584, 33.7058) -> (10.1092, 33.7058) centre (10.0838, 33.7058) ccw
  line L758 (18.8542, 17.5542) -> (19.1364, 17.78)
  line L759 (10.0838, 33.7058) -> (10.0838, 34.8742)
  arc A2451 (20.4332, 17.3744) -> (20.5208, 17.2825) centre (20.477, 17.3285) ccw
  arc A2452 (18.8542, 16.8275) -> (18.8542, 16.7005) centre (18.8542, 16.764) ccw
  line L760 (45.8164, 23.0505) -> (46.1339, 23.3045)
  arc A2453 (46.9594, 22.1932) -> (46.9594, 22.1298) centre (46.9594, 22.1615) ccw
  line L761 (19.1364, 17.78) -> (19.1364, 16.764)
  arc A2454 (20.5616, 17.526) -> (20.3076, 17.78) centre (20.3076, 17.526) ccw
  arc A2455 (18.0199, 16.7005) -> (18.0199, 16.8275) centre (18.0199, 16.764) ccw
  arc A2456 (11.1559, 34.6344) -> (11.1876, 34.5947) centre (11.1717, 34.6146) ccw
  arc A2457 (46.4514, 22.1298) -> (46.4514, 22.1932) centre (46.4514, 22.1615) ccw
  arc A2458 (18.0199, 16.764) -> (18.2457, 16.9898) centre (18.0199, 16.9898) ccw
  line L762 (19.9972, 16.764) -> (20.5616, 16.764)
  arc A2459 (31.9018, 35.7307) -> (31.8522, 35.7703) centre (31.877, 35.7505) ccw
  arc A2460 (47.3086, 23.3045) -> (47.2451, 23.3045) centre (47.2769, 23.3045) ccw
  line L763 (47.2769, 23.3045) -> (47.2769, 22.1615)
  arc A2461 (45.8164, 22.1932) -> (45.8164, 22.1298) centre (45.8164, 22.1615) ccw
  arc A2462 (47.5944, 22.1298) -> (47.5944, 22.1932) centre (47.5944, 22.1615) ccw
  line L764 (18.2457, 17.78) -> (18.2457, 16.9898)
  arc A2463 (46.9395, 23.0753) -> (46.9792, 23.0257) centre (46.9594, 23.0505) ccw
  arc A2464 (20.4981, 17.526) -> (20.6251, 17.526) centre (20.5616, 17.526) ccw
  arc A2465 (46.1656, 23.3045) -> (46.1021, 23.3045) centre (46.1339, 23.3045) ccw
  line L765 (18.8542, 16.764) -> (19.4186, 16.764)
  arc A2466 (47.2967, 23.2797) -> (47.257, 23.3293) centre (47.2769, 23.3045) ccw
  arc A2467 (45.0215, 22.1298) -> (45.0215, 22.1932) centre (45.0215, 22.1615) ccw
  line L766 (46.1339, 23.3045) -> (46.1339, 22.1615)
  line L767 (46.9594, 23.0505) -> (47.2769, 23.3045)
  arc A2468 (20.3076, 17.7165) -> (20.3076, 17.8435) centre (20.3076, 17.78) ccw
  arc A2469 (20.3076, 17.8435) -> (20.3076, 17.7165) centre (20.3076, 17.78) ccw
  arc A2470 (11.5122, 34.8544) -> (11.4804, 34.894) centre (11.4963, 34.8742) ccw
  arc A2471 (11.1718, 33.7312) -> (11.1718, 33.6804) centre (11.1718, 33.7058) ccw
  arc A2472 (11.8209, 33.6804) -> (11.8209, 33.7312) centre (11.8209, 33.7058) ccw
  line L768 (4.4958, 8.0518) -> (3.9878, 8.0518)
  arc A2473 (12.3825, 8.0328) -> (12.3825, 8.0963) centre (12.3825, 8.0646) ccw
  arc A2474 (4.4958, 8.02) -> (4.4958, 8.0836) centre (4.4958, 8.0518) ccw
  arc A2475 (3.5052, 8.02) -> (3.5052, 8.0836) centre (3.5052, 8.0518) ccw
  line L769 (4.9759, 9.1948) -> (5.2934, 9.1948)
  arc A2476 (5.5791, 8.8773) -> (5.6426, 8.8773) centre (5.6108, 8.8773) ccw
  arc A2477 (3.029, 9.1948) -> (2.9655, 9.1948) centre (2.9973, 9.1948) ccw
  arc A2478 (2.9972, 8.0836) -> (2.9972, 8.02) centre (2.9972, 8.0518) ccw
  line L770 (10.7329, 34.8742) -> (10.0838, 34.1602)
  arc A2479 (10.7517, 34.8571) -> (10.7141, 34.8913) centre (10.7329, 34.8742) ccw
  arc A2480 (6.4427, 8.0518) -> (6.5062, 8.0518) centre (6.4745, 8.0518) ccw
  arc A2481 (5.2934, 9.1631) -> (5.2934, 9.2266) centre (5.2934, 9.1949) ccw
  line L771 (5.2934, 8.0518) -> (4.9759, 8.0518)
  line L772 (3.9878, 8.0518) -> (3.9878, 9.1948)
  arc A2482 (5.2934, 8.0518) -> (5.6109, 8.3693) centre (5.2934, 8.3693) ccw
  arc A2483 (6.1371, 8.9656) -> (6.1768, 8.916) centre (6.157, 8.9408) ccw
  line L773 (6.157, 8.9408) -> (6.4745, 9.1948)
  arc A2484 (6.792, 8.02) -> (6.792, 8.0836) centre (6.792, 8.0518) ccw
  arc A2485 (5.6426, 8.3693) -> (5.5791, 8.3693) centre (5.6108, 8.3693) ccw
  line L774 (6.4745, 9.1948) -> (6.4745, 8.0518)
  line L775 (5.6109, 8.8773) -> (5.6109, 8.3693)
  arc A2486 (5.2934, 8.0836) -> (5.2934, 8.02) centre (5.2934, 8.0518) ccw
  arc A2487 (10.065, 34.1773) -> (10.1026, 34.1431) centre (10.0838, 34.1602) ccw
  arc A2488 (2.9655, 8.0518) -> (3.029, 8.0518) centre (2.9973, 8.0518) ccw
  arc A2489 (5.5791, 8.3693) -> (5.6426, 8.3693) centre (5.6108, 8.3693) ccw
  line L776 (3.9878, 8.6868) -> (4.3688, 8.6868)
  arc A2490 (5.6426, 8.8773) -> (5.5791, 8.8773) centre (5.6108, 8.8773) ccw
  arc A2491 (10.7106, 33.6936) -> (10.7552, 33.718) centre (10.7329, 33.7058) ccw
  line L777 (11.1718, 34.6146) -> (11.4963, 34.8742)
  line L778 (6.157, 8.0518) -> (6.792, 8.0518)
  arc A2492 (15.6693, 8.0328) -> (15.6693, 8.0963) centre (15.6693, 8.0646) ccw
  arc A2493 (3.956, 8.0518) -> (4.0195, 8.0518) centre (3.9878, 8.0518) ccw
  line L779 (11.8745, 9.2075) -> (11.8745, 8.0645)
  arc A2494 (5.2934, 9.2266) -> (5.2934, 9.1631) centre (5.2934, 9.1949) ccw
  arc A2495 (6.157, 8.0836) -> (6.157, 8.02) centre (6.157, 8.0518) ccw
  arc A2496 (3.9878, 8.0836) -> (3.9878, 8.02) centre (3.9878, 8.0518) ccw
  line L780 (2.9972, 8.0518) -> (3.5052, 8.0518)
  line L781 (3.9878, 9.1948) -> (4.4958, 9.1948)
  arc A2497 (4.4958, 9.1631) -> (4.4958, 9.2266) centre (4.4958, 9.1949) ccw
  arc A2498 (5.2934, 8.02) -> (5.2934, 8.0836) centre (5.2934, 8.0518) ccw
  arc A2499 (4.0195, 9.1948) -> (3.956, 9.1948) centre (3.9878, 9.1948) ccw
  arc A2500 (3.9878, 9.2266) -> (3.9878, 9.1631) centre (3.9878, 9.1949) ccw
  line L782 (11.4963, 34.8742) -> (11.4963, 33.7058)
  arc A2501 (4.3688, 8.655) -> (4.3688, 8.7186) centre (4.3688, 8.6868) ccw
  line L783 (4.9759, 8.0518) -> (4.9759, 9.1948)
  arc A2502 (11.5217, 34.8742) -> (11.4709, 34.8742) centre (11.4963, 34.8742) ccw
  arc A2503 (4.9759, 9.2266) -> (4.9759, 9.1631) centre (4.9759, 9.1949) ccw
  arc A2504 (4.9759, 8.0836) -> (4.9759, 8.02) centre (4.9759, 8.0518) ccw
  arc A2505 (3.9878, 8.7186) -> (3.9878, 8.655) centre (3.9878, 8.6868) ccw
  arc A2506 (6.4943, 9.17) -> (6.4546, 9.2196) centre (6.4745, 9.1948) ccw
  arc A2507 (10.3657, 34.432) -> (10.3211, 34.4077) centre (10.3434, 34.4199) ccw
  line L784 (13.3731, 8.0645) -> (12.8651, 8.0645)
  arc A2508 (5.6109, 8.8773) -> (5.2934, 9.1948) centre (5.2934, 8.8773) ccw
  arc A2509 (15.701, 8.9218) -> (15.6375, 8.9217) centre (15.6692, 8.9218) ccw
  arc A2510 (6.5062, 9.1948) -> (6.4427, 9.1948) centre (6.4745, 9.1948) ccw
  arc A2511 (5.0076, 9.1948) -> (4.9441, 9.1948) centre (4.9759, 9.1948) ccw
  arc A2512 (4.9441, 8.0518) -> (5.0076, 8.0518) centre (4.9759, 8.0518) ccw
  line L785 (2.9972, 9.1948) -> (2.9972, 8.0518)
  arc A2513 (12.8968, 9.2075) -> (12.8333, 9.2075) centre (12.8651, 9.2075) ccw
  arc A2514 (14.1707, 9.1757) -> (14.1707, 9.2393) centre (14.1707, 9.2075) ccw
  arc A2515 (14.4564, 8.89) -> (14.5199, 8.89) centre (14.4881, 8.89) ccw
  line L786 (76.708, 14.5415) -> (76.3905, 14.5415)
  arc A2516 (15.0101, 8.0851) -> (15.0584, 8.0439) centre (15.0343, 8.0645) ccw
  arc A2517 (76.3905, 14.5733) -> (76.3905, 14.5098) centre (76.3905, 14.5416) ccw
  arc A2518 (14.1707, 9.2393) -> (14.1707, 9.1757) centre (14.1707, 9.2075) ccw
  arc A2519 (13.8214, 8.0645) -> (13.8849, 8.0645) centre (13.8532, 8.0645) ccw
  arc A2520 (14.1707, 8.0963) -> (14.1707, 8.0328) centre (14.1707, 8.0646) ccw
  arc A2521 (12.8651, 9.2393) -> (12.8651, 9.1757) centre (12.8651, 9.2075) ccw
  arc A2522 (77.5054, 14.9473) -> (77.545, 14.8977) centre (77.5252, 14.9225) ccw
  line L787 (77.5252, 14.9225) -> (77.8427, 15.1765)
  arc A2523 (76.3588, 14.0335) -> (76.4223, 14.0335) centre (76.3906, 14.0335) ccw
  line L788 (15.574, 8.6995) -> (15.0343, 8.0645)
  arc A2524 (13.3731, 9.1757) -> (13.3731, 9.2393) centre (13.3731, 9.2075) ccw
  arc A2525 (14.4564, 8.382) -> (14.5199, 8.382) centre (14.4881, 8.382) ccw
  arc A2526 (13.8532, 8.0963) -> (13.8532, 8.0328) centre (13.8532, 8.0646) ccw
  arc A2527 (76.3905, 15.2083) -> (76.3905, 15.1448) centre (76.3905, 15.1766) ccw
  line L789 (76.3905, 15.1765) -> (76.708, 15.1765)
  arc A2528 (76.7999, 14.5557) -> (76.7431, 14.5273) centre (76.7715, 14.5415) ccw
  arc A2529 (76.708, 15.1448) -> (76.708, 15.2083) centre (76.708, 15.1766) ccw
  line L790 (13.8532, 9.2075) -> (14.1707, 9.2075)
  line L791 (14.4882, 8.89) -> (14.4882, 8.382)
  line L792 (12.8651, 9.2075) -> (13.3731, 9.2075)
  arc A2530 (15.5521, 8.7225) -> (15.5959, 8.6765) centre (15.574, 8.6995) ccw
  line L793 (11.8745, 8.0645) -> (12.3825, 8.0645)
  arc A2531 (15.3835, 9.2075) -> (15.0343, 8.9535) centre (15.3835, 8.8404) ccw
  arc A2532 (12.8651, 8.0963) -> (12.8651, 8.0328) centre (12.8651, 8.0646) ccw
  line L794 (12.8651, 8.0645) -> (12.8651, 9.2075)
  arc A2533 (14.1707, 8.0328) -> (14.1707, 8.0963) centre (14.1707, 8.0646) ccw
  arc A2534 (11.9063, 9.2075) -> (11.8428, 9.2075) centre (11.8746, 9.2075) ccw
  arc A2535 (76.708, 14.5098) -> (76.708, 14.5733) centre (76.708, 14.5416) ccw
  arc A2536 (14.5199, 8.89) -> (14.4564, 8.89) centre (14.4881, 8.89) ccw
  arc A2537 (11.8428, 8.0645) -> (11.9063, 8.0645) centre (11.8746, 8.0645) ccw
  arc A2538 (15.3835, 9.1757) -> (15.3835, 9.2393) centre (15.3835, 9.2075) ccw
  arc A2539 (12.8333, 8.0645) -> (12.8968, 8.0645) centre (12.8651, 8.0645) ccw
  arc A2540 (77.8745, 15.1765) -> (77.811, 15.1765) centre (77.8428, 15.1765) ccw
  arc A2541 (14.4882, 8.89) -> (14.1707, 9.2075) centre (14.1707, 8.89) ccw
  arc A2542 (15.6375, 8.9218) -> (15.701, 8.9218) centre (15.6693, 8.9218) ccw
  arc A2543 (13.8849, 9.2075) -> (13.8214, 9.2075) centre (13.8532, 9.2075) ccw
  arc A2544 (15.3835, 9.2393) -> (15.3835, 9.1757) centre (15.3835, 9.2075) ccw
  line L795 (14.1707, 8.0645) -> (13.8532, 8.0645)
  line L796 (77.5252, 14.0335) -> (78.1602, 14.0335)
  arc A2545 (14.1707, 8.0645) -> (14.4882, 8.382) centre (14.1707, 8.382) ccw
  arc A2546 (78.1602, 14.0017) -> (78.1602, 14.0653) centre (78.1602, 14.0335) ccw
  arc A2547 (15.574, 8.6995) -> (15.6693, 8.9218) centre (15.3624, 8.9218) ccw
  arc A2548 (11.8745, 8.0963) -> (11.8745, 8.0328) centre (11.8745, 8.0646) ccw
  arc A2549 (15.0343, 8.0963) -> (15.0343, 8.0328) centre (15.0343, 8.0646) ccw
  arc A2550 (15.6693, 8.9218) -> (15.3835, 9.2075) centre (15.3835, 8.9217) ccw
  line L797 (12.8651, 8.6995) -> (13.2461, 8.6995)